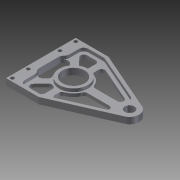
# Autodesk Inventor part: lower bix side plate 4
Saved by Autodesk Inventor 2012 (Build 160160000, 160)
## iProperties
Created: 2012-12-28
Part Number: lower bix side plate 4
Material: Default
Document SubType Name: Modeling
Designer: Bryce
Density: 1 g/cm^3
Author: Bryce
Autodesk Inventor part; units mm, degrees
ref_plane "YZ Plane" through (0, 0, 0) normal (1, 0, 0) x (0, 1, 0)
ref_plane "XZ Plane" through (0, 0, 0) normal (0, 1, 0) x (-1, 0, 0)
ref_plane "XY Plane" through (0, 0, 0) normal (0, 0, 1) x (1, 0, 0)
sketch "Sketch1" plane through (0, 0, 0) normal (0, 0, 1) x (1, 0, 0)
  line L0 (-34.925, 88.9) -> (34.925, 88.9)
  line L1 (34.925, 88.9) -> (34.925, 56.1594)
  line L2 (-34.925, 56.1594) -> (-34.925, 88.9)
  line L3 (-34.925, 56.1594) -> (-8.7286, -3.8127)
  line L4 (34.925, 56.1594) -> (8.7286, -3.8127)
  arc A0 (-8.7286, -3.8127) -> (8.7286, -3.8127) centre (0, 0) ccw
  circle A1 centre (0, 0) radius 4.7625
  circle A2 centre (0, 56.1594) radius 11.1125
  line L5 (0, 56.1594) -> (-34.925, 56.1594) construction
  line L6 (0, 56.1594) -> (34.925, 56.1594) construction
  line L7 (0, 56.1594) -> (-34.925, 88.9) construction
  line L8 (0, 56.1594) -> (34.925, 88.9) construction
  line L9 (0, 56.1594) -> (0, 0) construction
  line L10 (0, 56.1594) -> (0, 0) construction
  arc A3 (-15.5543, 52.9844) -> (-3.9688, 40.7885) centre (0, 56.1594) ccw
  arc A4 (3.9688, 40.7885) -> (15.5543, 52.9844) centre (0, 56.1594) ccw
  arc A5 (15.5543, 59.3344) -> (13.5191, 64.481) centre (0, 56.1594) ccw
  arc A6 (9.1762, 69.1137) -> (-9.1762, 69.1137) centre (0, 56.1594) ccw
  arc A7 (-13.5191, 64.481) -> (-15.5543, 59.3344) centre (0, 56.1594) ccw
  line L11 (-3.9688, 40.7885) -> (-3.9688, 8.6588)
  line L12 (3.9688, 40.7885) -> (3.9688, 8.6588)
  arc A8 (-3.9688, 8.6588) -> (-6.5042, 6.9585) centre (0, 0) ccw
  arc A9 (6.5042, 6.9585) -> (3.9688, 8.6588) centre (0, 0) ccw
  line L13 (-26.6088, 52.9844) -> (-6.5042, 6.9585)
  line L14 (6.5042, 6.9585) -> (26.6088, 52.9844)
  line L15 (-26.6088, 52.9844) -> (-15.5543, 52.9844)
  line L16 (-28.575, 59.3344) -> (-15.5543, 59.3344)
  line L17 (15.5543, 52.9844) -> (26.6088, 52.9844)
  line L18 (15.5543, 59.3344) -> (28.575, 59.3344)
  line L19 (-28.575, 78.5952) -> (-13.5191, 64.481)
  line L20 (-21.8156, 80.9625) -> (-9.1762, 69.1137)
  line L21 (21.8156, 80.9625) -> (9.1762, 69.1137)
  line L22 (28.575, 78.5952) -> (13.5191, 64.481)
  line L23 (-28.575, 78.5952) -> (-28.575, 59.3344)
  line L24 (-21.8156, 80.9625) -> (21.8156, 80.9625)
  line L25 (28.575, 78.5952) -> (28.575, 59.3344)
  arc A10 (3.9688, 16.3544) -> (10.0533, 15.0835) centre (7.1437, 16.3544) ccw
  arc A11 (-10.0533, 15.0835) -> (-3.9687, 16.3544) centre (-7.1437, 16.3544) ccw
  point P0 (-31.75, 85.725)
  point P1 (31.75, 85.725)
  point P2 (-15.875, 85.725)
  point P3 (15.875, 85.725)
  dimension "d0" = 69.85
  dimension "d1" = 88.9
  dimension "d2" = 34.925
  dimension "d6" = 23.596
  dimension "d7" = 9.525
  dimension "d8" = 32.7406
  dimension "d9" = 22.225
  dimension "d12" = 15.875
  dimension "d13" = 3.9688
  dimension "d14" = 3.9688
  dimension "d15" = 6.35
  dimension "d16" = 6.35
  dimension "d17" = 3.175
  dimension "d18" = 3.175
  dimension "d19" = 3.175
  dimension "d20" = 3.175
  dimension "d21" = 3.175
  dimension "d22" = 3.175
  dimension "d24" = 3.175
  dimension "d25" = 3.175
  dimension "d26" = 6.35
  dimension "d27" = 7.9375
  dimension "d28" = 6.35
  dimension "d32" = 3.175
  dimension "d33" = 3.175
  dimension "d35" = 3.175
  dimension "d36" = 3.175
  dimension "d62" = 19.05
  dimension "d63" = 19.05
  dimension "d69" = 3.175
  dimension "d70" = 23.596
  dimension "d71" = 9.525
  constraints: 52 end point, 20 point on circle, 13 parallel, 12 centre point, 9 coincident, 7 equal radius, 7 perpendicular, 5 tangent, 4 horizontal alignment, 4 point on line, 1 collinear, 1 horizontal, 1 vertical alignment
  measures "d0" distance between parallel lines of L1 L2
  measures "d1" distance from line of point (0, 0) L0
  measures "d2" distance from line of point (0, 0) L2
  measures "d6" angle of L1 L4
  measures "d7" diameter of A1
  measures "d8" distance from line of L5.start L0
  measures "d9" diameter of A2
  measures "d12" radius of A3
  measures "d13" distance between parallel lines of L9 L11
  measures "d14" distance between parallel lines of L9 L12
  measures "d15" distance between parallel lines of L3 L13
  measures "d16" distance between parallel lines of L4 L14
  measures "d17" distance between parallel lines of L15 L5
  measures "d18" distance between parallel lines of L5 L16
  measures "d19" distance between parallel lines of L17 L6
  measures "d20" distance between parallel lines of L6 L18
  measures "d21" distance between parallel lines of L8 L21
  measures "d22" distance between parallel lines of L8 L22
  measures "d24" distance between parallel lines of L7 L19
  measures "d25" distance between parallel lines of L7 L20
  measures "d26" distance between parallel lines of L23 L2
  measures "d27" distance between parallel lines of L0 L24
  measures "d28" distance between parallel lines of L1 L25
  measures "d32" distance from line of L2 point (-31.75, 85.725)
  measures "d33" distance from line of L0 point (-31.75, 85.725)
  measures "d35" distance from line of L0 point (31.75, 85.725)
  measures "d36" distance from line of L1 point (31.75, 85.725)
  measures "d62" distance from line of L2 point (-15.875, 85.725)
  measures "d63" distance from line of point (15.875, 85.725) L1
  measures "d69" radius of A11
  measures "d70" angle of L3 L2
  measures "d71" radius of A0
extrude "Extrusion1" add sketch "Sketch1" against normal blind 3.175 contours L0 L1 L4 A0 L3 L2 | A3 L11 A11 L13 L15 | L11 A8 L13 A11 | A4 L17 L14 A10 L12 | A10 L14 A9 L12 | A5 L22 L25 L18 | A6 L20 L24 L21 | A7 L16 L23 L19
extrude "Extrusion2" cut sketch "Sketch1" against normal blind 3.175 contours A3 L11 A11 L13 L15 | A4 L17 L14 A10 L12 | A5 L22 L25 L18 | A6 L20 L24 L21 | A7 L16 L23 L19
fillet "Fillet1" radius 3.175 16 edges at (-28.575, 59.3344, -1.5875) (-28.575, 78.5952, -1.5875) (28.575, 78.5952, -1.5875) (28.575, 59.3344, -1.5875) (15.5543, 59.3344, -1.5875) (13.5191, 64.481, -1.5875) (9.1762, 69.1137, -1.5875) (-9.1762, 69.1137, -1.5875) (-13.5191, 64.481, -1.5875) (-15.5543, 59.3344, -1.5875) (15.5543, 52.9844, -1.5875) (26.6088, 52.9844, -1.5875) (3.9687, 40.7885, -1.5875) (-3.9688, 40.7885, -1.5875) (-15.5543, 52.9844, -1.5875) (-26.6088, 52.9844, -1.5875)
hole "Hole1" at (-31.75, 85.725, 0) at (31.75, 85.725, 0) at (-15.875, 85.725, 0) at (15.875, 85.725, 0) direction (0, 0, -1) diameter 3.6576 end through all
sketch "Sketch2" plane through (0, 0, 0) normal (0, 0, 1) x (1, 0, 0)
  circle A0 centre (31.75, 85.725) radius 1.8288 projected
  circle A1 centre (-31.75, 85.725) radius 1.8288 projected
  line L0 (21.8156, 80.9625) -> (10.9317, 70.7593) projected
  arc A2 (7.3002, 70.2563) -> (10.9317, 70.7593) centre (8.7602, 73.0757) ccw projected
  arc A3 (7.3002, 70.2563) -> (-7.3002, 70.2563) centre (0, 56.1594) ccw projected
  arc A4 (-10.9317, 70.7593) -> (-7.3002, 70.2563) centre (-8.7602, 73.0757) ccw projected
  line L1 (-10.9317, 70.7593) -> (-21.8156, 80.9625) projected
  line L2 (-21.8156, 80.9625) -> (21.8156, 80.9625) projected
  circle A5 centre (0, 56.1594) radius 11.1125 projected
  circle A6 centre (0, 0) radius 4.7625 projected
  line L3 (-34.925, 56.1594) -> (-34.925, 88.9) projected
  line L4 (-8.7286, -3.8127) -> (-34.925, 56.1594) projected
  arc A7 (-8.7286, -3.8127) -> (8.7286, -3.8127) centre (0, 0) ccw projected
  line L5 (34.925, 56.1594) -> (8.7286, -3.8127) projected
  line L6 (34.925, 88.9) -> (34.925, 56.1594) projected
  line L7 (-34.925, 88.9) -> (34.925, 88.9)
  line L8 (34.925, 88.9) -> (34.925, 77.7875)
  line L9 (34.925, 77.7875) -> (31.75, 77.7875) construction
  line L10 (-34.925, 77.7875) -> (-34.925, 88.9)
  line L11 (-18.4288, 77.7875) -> (-31.75, 77.7875)
  line L12 (18.4288, 77.7875) -> (-18.4288, 77.7875) construction
  line L13 (-31.75, 77.7875) -> (-31.75, 56.8226)
  line L14 (-31.75, 56.8226) -> (-8.6609, 3.9641)
  line L15 (31.75, 77.7875) -> (31.75, 56.8226)
  line L16 (31.75, 56.8226) -> (8.6609, 3.9641)
  arc A8 (0, 9.525) -> (-8.6609, 3.9641) centre (0, 0) ccw
  arc A9 (8.6609, 3.9641) -> (0, 9.525) centre (0, 0) ccw
  line L17 (0, 56.1594) -> (0, 0) construction
  line L18 (-31.75, 77.7875) -> (-34.925, 77.7875) construction
  line L19 (31.75, 77.7875) -> (18.4288, 77.7875)
  circle A10 centre (15.875, 85.725) radius 1.8288 projected
  circle A11 centre (-15.875, 85.725) radius 1.8288 projected
  circle A12 centre (-15.875, 85.725) radius 1.8288
  circle A13 centre (15.875, 85.725) radius 1.8288
  arc A14 (-14.5384, 62.5352) -> (-14.9671, 61.4511) centre (0, 56.1594) ccw projected
  circle A15 centre (0, 56.1594) radius 14.2875
  dimension "d45" = 11.1125
  dimension "d46" = 3.175
  dimension "d47" = 3.175
  dimension "d48" = 3.175
  dimension "d49" = 3.175
  dimension "d53" = 22.225
  dimension "d72" = 28.575
  constraints: 26 end point, 9 parallel, 6 coincident, 5 centre point, 4 concentric, 4 point on circle, 4 point on line, 2 perpendicular, 1 horizontal
  measures "d45" distance between parallel lines of L9 L7
  measures "d46" distance between parallel lines of L3 L13
  measures "d47" distance between parallel lines of L4 L14
  measures "d48" distance between parallel lines of L5 L16
  measures "d49" distance between parallel lines of L6 L15
  measures "d53" diameter of A5
  measures "d72" diameter of A15
extrude "Extrusion4" add sketch "Sketch2" along normal blind 3.175
fillet "Fillet6" radius 4.7625 8 edges at (-21.8156, 80.9625, 0) (-31.75, 77.7875, 1.5875) (-31.75, 56.8226, 1.5875) (31.75, 77.7875, 1.5875) (21.8156, 80.9625, 0) (31.75, 56.8226, 1.5875) (-8.6609, 3.9641, 1.5875) (8.6609, 3.9641, 1.5875)
fillet "Fillet8" radius 6.35 2 edges at (-14.262, 77.7875, 1.5875) (14.262, 77.7875, 1.5875)
body "Solid1"
